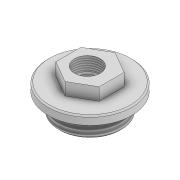
# Autodesk Inventor part: 螺盖
Saved by Autodesk Inventor 2022 (Build 260153000, 153)
## iProperties
Created: 2023-03-14
Part Number: 螺盖
Material: 常规
Document SubType Name: Modeling
Designer: Lzy18
Density: 1 g/cm^3
Appearance: 默认
Author: Lzy18
Autodesk Inventor part; units mm, degrees
ref_plane "YZ Plane" through (0, 0, 0) normal (1, 0, 0) x (0, 1, 0)
ref_plane "XZ Plane" through (0, 0, 0) normal (0, 1, 0) x (-1, 0, 0)
ref_plane "XY Plane" through (0, 0, 0) normal (0, 0, 1) x (1, 0, 0)
sketch "草图1" plane through (0, 0, 0) normal (0, 1, 0) x (-1, 0, 0)
  circle A0 centre (0, 0) radius 60
  dimension "d0" = 120
  constraints: 1 centre point, 1 coincident
  measures "d0" diameter of A0
extrude "拉伸1" add sketch "草图1" along normal mid plane 12
sketch "草图2" plane through (0, -6, 0) normal (0, -1, 0) x (1, 0, 0)
  circle A0 centre (0, 0) radius 41
  dimension "d3" = 82
  constraints: 1 centre point, 1 coincident
  measures "d3" diameter of A0
extrude "拉伸2" add sketch "草图2" along normal blind 3
sketch "草图3" plane through (0, -9, 0) normal (0, -1, 0) x (1, 0, 0)
  circle A0 centre (0, 0) radius 45
  dimension "d6" = 90
  constraints: 1 centre point, 1 coincident
  measures "d6" diameter of A0
extrude "拉伸3" add sketch "草图3" along normal blind 24
thread "螺纹1" size "M90x6" class "6g" standard "GB Metric profile" full length
sketch "草图4" plane through (0, 6, 0) normal (0, 1, 0) x (1, 0, 0)
  line L0 (-31, 17.8979) -> (0, 35.7957)
  line L1 (0, 35.7957) -> (31, 17.8979)
  line L2 (31, 17.8979) -> (31, -17.8979)
  line L3 (31, -17.8979) -> (0, -35.7957)
  line L4 (0, -35.7957) -> (-31, -17.8979)
  line L5 (-31, -17.8979) -> (-31, 17.8979)
  point P0 (0, 0)
  point P1 (0, 0)
  dimension "d11" = 62
  constraints: 12 end point, 1 coincident, 13 other
  measures "d11" distance between parallel lines of L2 L5
extrude "拉伸4" add sketch "草图4" along normal blind 18
sketch "草图5" plane through (0, 24, 0) normal (0, 1, 0) x (1, 0, 0)
  line L0 (0, 35.7957) -> (-31, 17.8979) projected
  point P0 (0, 0)
  point P1 (-3.1488, -0.6537)
  dimension "d14" = 29.9917
  measures "d14" distance from line of L0 point (-3.149, -0.654)
hole "孔1" at (-3.1488, 24, 0.6537) direction (0, -1, 0) diameter 36.7524 depth 20 thread size "M40x3" class "6H" standard "GB Metric profile"
sketch "草图6" plane through (-3.1488, 4, 0.6537) normal (0, 1, 0) x (1, 0, 0)
  circle A0 centre (0, 0) radius 18.3762 projected
  point P0 (3.1488, 0.6537)
  constraints: 1 coincident
hole "孔2" at (-3.1488, 4, 0.6537) direction (0, -1, 0) diameter 41 depth 5
sketch "草图7" plane through (-3.1488, -1, 0.6537) normal (0, 1, 0) x (1, 0, 0)
  circle A0 centre (0, 0) radius 20.5 projected
  point P0 (3.1488, 0.6537)
  constraints: 1 coincident
hole "孔3" at (-3.1488, -1, 0.6537) direction (0, -1, 0) diameter 22 depth 5
sketch "草图8" plane through (-3.1488, -6, 0.6537) normal (0, 1, 0) x (1, 0, 0)
  circle A0 centre (0, 0) radius 11 projected
  point P0 (3.1488, 0.6537)
  constraints: 1 coincident
hole "孔4" at (-3.1488, -6, 0.6537) direction (0, -1, 0) diameter 45.6699 end through all thread size "M50x4" class "6H" standard "GB Metric profile"
chamfer "倒角1" distance 2 angle 45 2 edges at (60, 6, 0) (-45, -33, 0)
